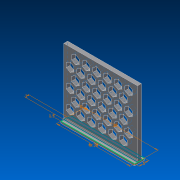
# Autodesk Inventor part: vent test hex 2
Saved by Autodesk Inventor 2015 (Build 190159000, 159)
## iProperties
Created: 2017-03-16
Part Number: vent test hex 2
Material: Generic
Document SubType Name: Modeling
Designer: ZigZagJoe
Density: 1 g/cm^3
Appearance: Default
Author: ZigZagJoe
Autodesk Inventor part; units mm, degrees
ref_plane "YZ Plane" through (0, 0, 0) normal (1, 0, 0) x (0, 1, 0)
ref_plane "XZ Plane" through (0, 0, 0) normal (0, 1, 0) x (-1, 0, 0)
ref_plane "XY Plane" through (0, 0, 0) normal (0, 0, 1) x (1, 0, 0)
sketch "Sketch1" plane through (0, 0, 0) normal (0, 0, 1) x (1, 0, 0)
  line L0 (-19.4684, -0.3877) -> (18.5316, -0.3877)
  line L1 (18.5316, -0.3877) -> (18.5316, -5.3877)
  line L2 (18.5316, -5.3877) -> (-19.4684, -5.3877)
  line L3 (-19.4684, -5.3877) -> (-19.4684, -0.3877)
  line L4 (-19.4684, -1.8877) -> (18.5316, -1.8877)
  line L5 (18.5316, -1.8877) -> (18.5316, -3.8877)
  line L6 (18.5316, -3.8877) -> (-19.4684, -3.8877)
  line L7 (-19.4684, -3.8877) -> (-19.4684, -1.8877)
  point P0 (0, 0)
  dimension "d0" = 38
  dimension "d1" = 5
  dimension "d4" = 2
  dimension "d5" = 38
  dimension "d7" = 1.5
  dimension "d56" = 0
  constraints: 16 end point, 4 parallel, 2 horizontal, 2 perpendicular
  measures "d0" distance of L1.end L2.end
  measures "d1" distance of L0.end L1.end
  measures "d4" distance of L6.end L4.start
  measures "d5" distance of L4.start L4.end
  measures "d7" distance between parallel lines of L2 L6
  measures "d56" distance between parallel lines of L3 L7
extrude "Extrusion1" add sketch "Sketch1" along normal blind 34 contours L4 L1 L6 L3
extrude "Extrusion2" add sketch "Sketch1" against normal blind 1
fillet "Fillet1" radius 1 2 edges at (-0.4684, -3.8877, 0) (-0.4684, -1.8877, 0)
sketch "Sketch2" plane through (-19.4684, -3.8877, 34) normal (0, -1, 0) x (1, 0, 0)
  line L0 (37, -1) -> (1, -1)
  line L1 (1, -1) -> (1, -17)
  line L2 (1, -17) -> (37, -17)
  line L3 (37, -17) -> (37, -1)
  line L4 (0, 0) -> (38, 0) projected
  line L5 (2.3536, -1) -> (7.3536, -1) construction
  line L6 (8.0711, -1) -> (5.2426, -3.8284)
  line L7 (5.2426, -3.8284) -> (2.4142, -1)
  line L8 (1, -2.4142) -> (3.8284, -5.2426)
  line L9 (3.8284, -5.2426) -> (1, -8.0711)
  line L10 (1, -8.0711) -> (2.4142, -9.4853)
  line L11 (2.4142, -9.4853) -> (5.2426, -6.6569)
  line L12 (5.2426, -6.6569) -> (8.0711, -9.4853)
  line L13 (8.0711, -9.4853) -> (9.4853, -8.0711)
  line L14 (9.4853, -8.0711) -> (6.6569, -5.2426)
  line L15 (6.6569, -5.2426) -> (9.4853, -2.4142)
  line L16 (9.4853, -2.4142) -> (8.0711, -1)
  line L17 (2.4142, -1) -> (1, -2.4142)
  line L18 (9.4853, -2.4142) -> (9.4853, -8.0711)
  line L19 (8.0711, -9.4853) -> (2.4142, -9.4853)
  line L20 (1, -8.0711) -> (1, -2.4142)
  line L21 (2.4142, -1) -> (8.0711, -1)
  line L22 (38, -33) -> (38, 0) projected
  line L23 (0, -33) -> (0, 0) projected
  point P0 (19.4684, -34)
  dimension "d28" = 4
  dimension "d29" = 2
  dimension "d30" = 4
  dimension "d31" = 2
  dimension "d32" = 4
  dimension "d39" = 8.4853
  dimension "d40" = 1
  dimension "d41" = 1
  dimension "d42" = 1
  constraints: 42 end point, 12 point on line, 7 perpendicular, 4 parallel, 2 horizontal, 1 collinear
  measures "d28" distance of L11.end L12.end
  measures "d29" distance of L12.end L13.end
  measures "d30" distance of L14.end L15.end
  measures "d31" distance between parallel lines of L11 L9
  measures "d32" distance of L8.start L8.end
  measures "d39" horizontal distance of L13.end L8.start
  measures "d40" distance between parallel lines of L22 L3
  measures "d41" distance between parallel lines of L23 L20
  measures "d42" distance between parallel lines of L4 L0
extrude "Extrusion3" [suppressed]
pattern_linear "Rectangular Pattern1" [suppressed]
sketch "Sketch3" plane through (-19.4684, -3.8877, 34) normal (0, -1, 0) x (1, 0, 0)
  line L0 (3, -3) -> (3, -21) construction
  line L1 (2, -3) -> (2, -21)
  line L2 (4, -21) -> (4, -3)
  arc A0 (4, -3) -> (2, -3) centre (3, -3) ccw
  arc A1 (2, -21) -> (4, -21) centre (3, -21) ccw
  line L3 (0, 0) -> (38, 0) projected
  line L4 (0, -33) -> (0, 0) projected
  point P0 (19.4684, -34)
  point P1 (3, -12)
  dimension "d43" = 2
  dimension "d44" = 3
  dimension "d45" = 18
  dimension "d48" = 3
  constraints: 8 end point, 4 point on circle, 4 tangent, 2 centre point, 1 midpoint, 1 parallel, 1 vertical
  measures "d43" diameter of A1
  measures "d44" distance from line of L0.start L3
  measures "d45" distance of L0.start L0.end
  measures "d48" distance from line of L4 L0.start
extrude "Extrusion4" [suppressed]
pattern_linear "Rectangular Pattern2" [suppressed]
fillet "Fillet2" [suppressed]
sketch "Sketch4" plane through (-19.4684, -3.8877, 34) normal (0, -1, 0) x (1, 0, 0)
  line L0 (6, -2) -> (8, -3.1547)
  line L1 (8, -3.1547) -> (8, -5.4641)
  line L2 (8, -5.4641) -> (6, -6.6188)
  line L3 (6, -6.6188) -> (4, -5.4641)
  line L4 (4, -5.4641) -> (4, -3.1547)
  line L5 (4, -3.1547) -> (6, -2)
  line L6 (0, -33) -> (0, 0) projected
  line L7 (5.25, -10.2272) -> (3.25, -11.3819)
  line L8 (3.25, -11.3819) -> (1.25, -10.2272)
  line L9 (1.25, -10.2272) -> (1.25, -7.9178)
  line L10 (1.25, -7.9178) -> (3.25, -6.7631)
  line L11 (3.25, -6.7631) -> (5.25, -7.9178)
  line L12 (5.25, -7.9178) -> (5.25, -10.2272)
  line L13 (10.75, -10.2272) -> (8.75, -11.3819)
  line L14 (8.75, -11.3819) -> (6.75, -10.2272)
  line L15 (6.75, -10.2272) -> (6.75, -7.9178)
  line L16 (6.75, -7.9178) -> (8.75, -6.7631)
  line L17 (8.75, -6.7631) -> (10.75, -7.9178)
  line L18 (10.75, -7.9178) -> (10.75, -10.2272)
  line L19 (13.5, -3.1547) -> (13.5, -5.4641)
  line L20 (13.5, -5.4641) -> (11.5, -6.6188)
  line L21 (11.5, -6.6188) -> (9.5, -5.4641)
  line L22 (9.5, -5.4641) -> (9.5, -3.1547)
  line L23 (9.5, -3.1547) -> (11.5, -2)
  line L24 (11.5, -2) -> (13.5, -3.1547)
  point P0 (19.4684, -34)
  point P1 (6, -4.3094)
  point P2 (3.25, -9.0725)
  point P3 (8.75, -9.0725)
  point P4 (11.5, -4.3094)
  dimension "d57" = 4
  dimension "d58" = 2
  dimension "d59" = 4
  dimension "d62" = 0
  dimension "d63" = 4
  dimension "d64" = 1.5
  dimension "d65" = 0.75
  dimension "d67" = 1.5
  dimension "d68" = 1.5
  dimension "d69" = 4
  dimension "d71" = 4
  dimension "d72" = 1.5
  dimension "d73" = 1.5
  dimension "d80" = 12.25
  dimension "d81" = 9.3819
  constraints: 48 end point, 52 other
  measures "d57" distance between parallel lines of L6 L4
  measures "d58" vertical distance of L6.end L0.start
  measures "d59" distance between parallel lines of L5 L2
  measures "d62" angle of L6 L9
  measures "d63" distance between parallel lines of L7 L10
  measures "d64" distance of L3.end L10.end
  measures "d65" horizontal distance of L11.end L2.end
  measures "d67" distance between parallel lines of L15 L12
  measures "d68" distance of L1.end L16.end
  measures "d69" distance between parallel lines of L13 L16
  measures "d71" distance between parallel lines of L20 L23
  measures "d72" distance between parallel lines of L21 L17
  measures "d73" distance of L22.end L0.end
  measures "d80" horizontal distance of L19.start L9.end
  measures "d81" vertical distance of L7.end L0.start
extrude "Extrusion5" cut sketch "Sketch4" against normal blind 10
pattern_linear "Rectangular Pattern3" count 3 spacing 11 along (1, 0, 0) count 3 spacing 9.5 along (0, 0, -1) of "Extrusion5"
equation "\"d0\" = d5"
equation "\"d28\" = d32"
equation "\"d29\" = d31"
equation "\"d30\" = d32"
equation "\"d57\" = d59"
equation "\"d63\" = d59"
equation "\"d65\" = 0.5 * d64"
equation "\"d67\" = d64"
equation "\"d68\" = d64"
equation "\"d69\" = d59"
equation "\"d71\" = d59"
equation "\"d72\" = d64"
equation "\"d73\" = d64"
body "Solid1"
